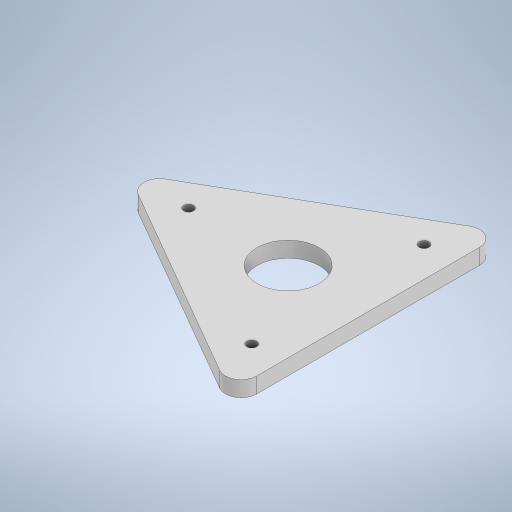
# Autodesk Inventor part: AP-1-01-planetCarrier
Saved by Autodesk Inventor 2023 (Build 270158000, 158)
## iProperties
Created: 2023-07-11
Part Number: AP-1-01-planetCarrier
Material: Generic
Document SubType Name: Modeling
Designer: t205b
Density: 1 g/cm^3
Appearance: Default
Author: t205b
Autodesk Inventor part; units mm, degrees
ref_plane "YZ Plane" through (0, 0, 0) normal (1, 0, 0) x (0, 1, 0)
ref_plane "XZ Plane" through (0, 0, 0) normal (0, 1, 0) x (-1, 0, 0)
ref_plane "XY Plane" through (0, 0, 0) normal (0, 0, 1) x (1, 0, 0)
sketch "Sketch1" plane through (0, 0, 0) normal (0, 1, 0) x (-1, 0, 0)
  line L0 (153.9793, -88.9) -> (0, 0)
  line L1 (0, 0) -> (0, -177.8)
  line L2 (0, -177.8) -> (153.9793, -88.9)
  circle A0 centre (51.3264, -88.9) radius 20
  line L3 (76.9897, -133.35) -> (61.3264, -106.2205) construction
  line L4 (76.9897, -44.45) -> (61.3264, -71.5795) construction
  line L5 (31.3264, -88.9) -> (0, -88.9) construction
  circle A1 centre (115.2355, -88.9) radius 3.175
  circle A2 centre (19.3719, -144.2469) radius 3.175
  circle A3 centre (19.3719, -33.5531) radius 3.175
  line L6 (19.3719, -144.2469) -> (51.3264, -88.9) construction
  line L7 (51.3264, -88.9) -> (115.2355, -88.9) construction
  line L8 (51.3264, -88.9) -> (19.3719, -33.5531) construction
  dimension "d0" = 177.8
  dimension "d1" = 40
  dimension "d2" = 102.6529
  dimension "d3" = 63.9091
  dimension "d4" = 6.35
  dimension "d5" = 120
  dimension "d6" = 120
  constraints: 18 end point, 6 equal length, 4 centre point, 3 line through centre, 3 midpoint, 3 point on circle, 2 equal radius, 2 perpendicular, 1 coincident, 1 horizontal, 1 vertical
  measures "d0" distance of L0.end L1.end
  measures "d1" diameter of A0
  measures "d2" distance of L1.end L6.end
  measures "d3" distance of L6.start L6.end
  measures "d4" diameter of A2
  measures "d5" angle of L6 L7
  measures "d6" angle of L8 L7
extrude "Extrusion1" add sketch "Sketch1" along normal blind 10
fillet "Fillet1" radius 10 3 edges at (0, 5, -177.8) (0, 5, 0) (-153.9793, 5, -88.9)
body "Solid1"
